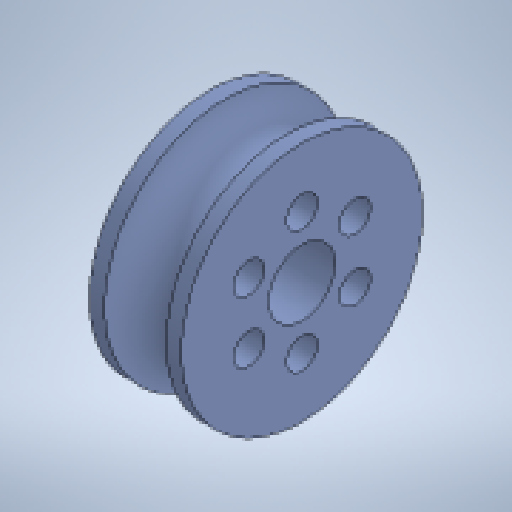
# Autodesk Inventor part: Idler - Puley
Saved by Autodesk Inventor 2023.2 (Build 272271000, 271)
## iProperties
Created: 2023-11-16
Part Number: Idler - Puley
Material: Nylon 6/6
Document SubType Name: Modeling
Designer: Nathan Cai
Density: 1.13 g/cm^3
Appearance: Rubber - Blue
Author: Nathan Cai
Autodesk Inventor part; units mm, degrees
ref_plane "YZ Plane" through (0, 0, 0) normal (1, 0, 0) x (0, 1, 0)
ref_plane "XZ Plane" through (0, 0, 0) normal (0, 1, 0) x (-1, 0, 0)
ref_plane "XY Plane" through (0, 0, 0) normal (0, 0, 1) x (1, 0, 0)
sketch "Sketch1" plane through (0, 0, 0) normal (0, 0, 1) x (1, 0, 0)
  line L0 (-4.7625, -12.5) -> (4.7625, -12.5)
  line L1 (4.7625, -12.5) -> (4.7625, 12.5)
  line L2 (4.7625, 12.5) -> (-4.7625, 12.5)
  line L3 (-4.7625, 12.5) -> (-4.7625, -12.5)
  line L4 (-4.7625, -12.5) -> (4.7625, 12.5) construction
  line L5 (4.7625, -12.5) -> (-4.7625, 12.5) construction
  circle A0 centre (0, 12.5) radius 3.175
  line L6 (-4.7625, -3.429) -> (4.7625, -3.429)
  line L7 (4.7625, -3.429) -> (4.7625, 3.429)
  line L8 (4.7625, 3.429) -> (-4.7625, 3.429)
  line L9 (-4.7625, 3.429) -> (-4.7625, -3.429)
  line L10 (-4.7625, -3.429) -> (4.7625, 3.429) construction
  line L11 (4.7625, -3.429) -> (-4.7625, 3.429) construction
  line L12 (-4.7625, 0) -> (4.7625, 0) construction
  point P0 (0, 0)
  point P1 (3.175, 12.5)
  point P2 (-3.175, 12.5)
  dimension "d0" = 9.525
  dimension "d1" = 25
  dimension "d2" = 6.35
  dimension "d3" = 9.525
  dimension "d4" = 6.858
  constraints: 26 end point, 7 midpoint, 4 parallel, 2 horizontal, 2 perpendicular, 1 centre point
  measures "d0" distance of L2.end L1.end
  measures "d1" distance of L1.end L0.end
  measures "d2" diameter of A0
  measures "d3" distance of L8.end L7.end
  measures "d4" distance of L7.end L6.end
revolve "Revolution1" add sketch "Sketch1" angle 360 about axis through (-4.7625, 0, 0) along (1, 0, 0) contours L3 L2 A0 L1 L8
sketch "Sketch2" plane through (4.7625, 0, 0) normal (1, 0, 0) x (0, 0, -1)
  circle A0 centre (0, 0) radius 6.35 construction
  line L0 (0, 6.35) -> (0, 0) construction
  circle A1 centre (0, 6.35) radius 1.5875
  circle A2 centre (-5.4993, 3.175) radius 1.5875
  circle A3 centre (-5.4993, -3.175) radius 1.5875
  circle A4 centre (0, -6.35) radius 1.5875
  circle A5 centre (5.4993, -3.175) radius 1.5875
  circle A6 centre (5.4993, 3.175) radius 1.5875
  dimension "d6" = 12.7
  dimension "d7" = 3.175
  dimension "d10" = 360
  constraints: 6 centre point, 2 coincident, 2 end point, 1 vertical, 1 vertical alignment, 15 other
  measures "d7" diameter of A1
extrude "Extrusion1" cut sketch "Sketch2" against normal through all
body "Solid1"
